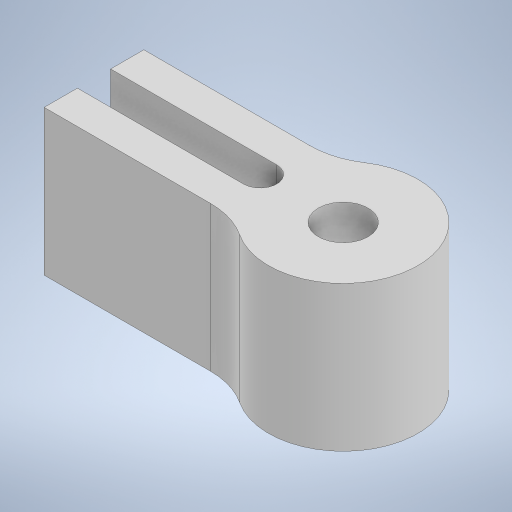
# Autodesk Inventor part: aperature clip
Saved by Autodesk Inventor 2024 (Build 280153000, 153)
## iProperties
Created: 2025-02-23
Part Number: aperature clip
Material: Generic
Document SubType Name: Modeling
Designer: Williamow
Density: 1 g/cm^3
Appearance: Default
Author: Williamow
Autodesk Inventor part; units mm, degrees
ref_plane "YZ Plane" through (0, 0, 0) normal (1, 0, 0) x (0, 1, 0)
ref_plane "XZ Plane" through (0, 0, 0) normal (0, 1, 0) x (-1, 0, 0)
ref_plane "XY Plane" through (0, 0, 0) normal (0, 0, 1) x (1, 0, 0)
sketch "Sketch2" plane through (0, 0, 0) normal (0, 1, 0) x (-1, 0, 0)
  circle A0 centre (0, 0) radius 0.6
  arc A1 (0.9908, 1.5028) -> (0.9908, -1.5028) centre (0, 0) ccw
  arc A2 (0.9908, 1.5028) -> (2, 1.2) centre (2, 3.0333) ccw
  arc A3 (2, -1.2) -> (0.9908, -1.5028) centre (2, -3.0333) ccw
  line L0 (2, 1.2) -> (6, 1.2)
  line L1 (6, 1.2) -> (6, 0.4)
  line L2 (6, 0.4) -> (2, 0.4)
  arc A4 (2, 0.4) -> (2, -0.4) centre (2, 0) ccw
  line L3 (2, -0.4) -> (6, -0.4)
  line L4 (6, -0.4) -> (6, -1.2)
  line L5 (6, -1.2) -> (2, -1.2)
  dimension "d7" = 1.2
  dimension "d8" = 1.2
  dimension "d9" = 0.8
  dimension "d10" = 0.8
  dimension "d11" = 6
  dimension "d12" = 2
  constraints: 12 end point, 8 point on circle, 5 centre point, 5 vertical alignment, 4 perpendicular, 4 tangent, 2 coincident, 2 horizontal, 1 equal radius, 1 horizontal alignment
  measures "d7" diameter of A0
  measures "d8" radial gap between concentric circles of A1 A0
  measures "d9" distance between parallel lines of L3 L2
  measures "d10" distance of L0.end L1.end
  measures "d11" distance from line of L1 point (0, 0)
  measures "d12" distance of point (0, 0) A4.centre
extrude "Extrusion2" add sketch "Sketch2" along normal blind 3.5
sketch "Sketch1" plane through (0, 0, 0) normal (0, 1, 0) x (-1, 0, 0)
  line L0 (0, -2) -> (0, 2)
  arc A0 (0, 2) -> (3, 1) centre (3, 6) ccw
  arc A1 (3, -1) -> (0, -2) centre (3, -6) ccw
  line L1 (0.8, 0.6334) -> (0.8, -0.6334)
  arc A2 (0.8, 0.6334) -> (3, 0.2) centre (3, 6) ccw
  arc A3 (3, -0.2) -> (0.8, -0.6334) centre (3, -6) ccw
  line L2 (3, 0.2) -> (3, 1)
  line L3 (3, -0.2) -> (3, -1)
  point P0 (0, 0)
  point P1 (0, 0)
  point P2 (0.8, 0)
  dimension "d0" = 4
  dimension "d1" = 0.8
  dimension "d2" = 0.8
  dimension "d3" = 0.4
  dimension "d4" = 3
  constraints: 8 end point, 8 point on circle, 4 centre point, 3 coincident, 3 vertical, 2 collinear, 2 midpoint, 1 horizontal alignment, 1 line through centre, 1 vertical alignment
  measures "d0" distance of L0.start L0.end
  measures "d1" radial gap between concentric circles of A2 A0
  measures "d2" distance between parallel lines of L0 L1
  measures "d3" distance of L3.start L2.start
  measures "d4" horizontal distance of L0.start L3.end
body "Solid1"
body "Solid2"
